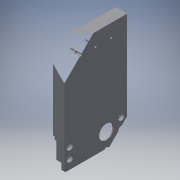
# Autodesk Inventor part: Base_motor_servo
Saved by Autodesk Inventor 2016 (Build 200138000, 138)
## iProperties
Created: 2018-05-05
Part Number: Base_motor_servo
Material: Genérico
Document SubType Name: Modeling
Designer: Innovacion Creativa
Density: 1 g/cm^3
Appearance: Valor por defecto
Author: Innovacion Creativa
Autodesk Inventor part; units mm, degrees
ref_plane "YZ Plane" through (0, 0, 0) normal (1, 0, 0) x (0, 1, 0)
ref_plane "XZ Plane" through (0, 0, 0) normal (0, 1, 0) x (-1, 0, 0)
ref_plane "XY Plane" through (0, 0, 0) normal (0, 0, 1) x (1, 0, 0)
sketch "Boceto2" plane through (0, 0, 0) normal (1, 0, 0) x (0, 1, 0)
  line L0 (44.4327, 14) -> (-16.1673, 14)
  line L1 (-16.1673, 14) -> (-16.1673, -14)
  line L2 (-16.1673, -14) -> (44.4327, -14)
  line L3 (44.4327, -14) -> (44.4327, 14)
  line L4 (-13.1673, 3.75) -> (-13.1673, -3.75) construction
  line L5 (41.4327, 3.75) -> (41.4327, -3.75) construction
  circle A0 centre (24.4327, 0) radius 6.4 construction
  circle A1 centre (24.4327, 0) radius 6.9
  point P0 (-16.1673, 0)
  point P1 (0, 0)
  dimension "d11" = 28
  dimension "d12" = 3
  dimension "d13" = 3
  dimension "d14" = 0.5
  constraints: 8 end point, 2 parallel, 1 centre point, 1 horizontal, 1 horizontal alignment, 1 midpoint, 1 perpendicular, 1 other
  measures "d11" distance of L0.end L1.end
  measures "d12" distance between parallel lines of L1 L4
  measures "d13" distance between parallel lines of L3 L5
  measures "d14" radial gap between concentric circles of A0 A1
extrude "Extrusión2" add sketch "Boceto2" along normal blind 1
sketch "Boceto3" plane through (0, 0, 0) normal (-1, 0, 0) x (0, 0, 1)
  line L0 (-8.9, 13.0341) -> (-1.9183, 13.0341) construction
  line L1 (-8.9, 1.5341) -> (-8.9, 13.0341) construction
  arc A0 (-8.9, 1.5341) -> (-7.9, 0.5341) centre (-7.9, 1.5341) ccw construction
  line L2 (7.9, 0.5341) -> (-7.9, 0.5341) construction
  arc A1 (7.9, 0.5341) -> (8.9, 1.5341) centre (7.9, 1.5341) ccw construction
  line L3 (8.9, 13.0341) -> (8.9, 1.5341) construction
  arc A2 (1.9183, 13.0341) -> (-1.9183, 13.0341) centre (0, 13.3841) ccw construction
  line L4 (1.9183, 13.0341) -> (8.9, 13.0341) construction
  line L5 (-8.9, 13.5341) -> (-2.8775, 13.5341)
  arc A3 (2.3898, 13.924) -> (-2.3898, 13.924) centre (0, 13.3841) ccw
  line L6 (2.8775, 13.5341) -> (8.9, 13.5341)
  line L7 (9.4, 13.0341) -> (9.4, 1.5341)
  arc A4 (7.9, 0.0341) -> (9.4, 1.5341) centre (7.9, 1.5341) ccw
  line L8 (7.9, 0.0341) -> (-7.9, 0.0341)
  arc A5 (-9.4, 1.5341) -> (-7.9, 0.0341) centre (-7.9, 1.5341) ccw
  line L9 (-9.4, 1.5341) -> (-9.4, 13.0341)
  arc A6 (-2.8775, 13.5341) -> (-2.3898, 13.924) centre (-2.8775, 14.0341) ccw
  arc A7 (2.3898, 13.924) -> (2.8775, 13.5341) centre (2.8775, 14.0341) ccw
  arc A8 (9.4, 13.0341) -> (8.9, 13.5341) centre (8.9, 13.0341) ccw
  arc A9 (-8.9, 13.5341) -> (-9.4, 13.0341) centre (-8.9, 13.0341) ccw
  point P0 (-2.4454, 13.5341)
  point P1 (2.4454, 13.5341)
  dimension "d19" = 0.5
  dimension "d20" = 0.5
  constraints: 16 point on circle, 10 end point, 8 tangent, 7 centre point, 3 equal radius, 2 point on line, 7 other
  measures "d19" distance between parallel lines of L1 L9
  measures "d20" radius of A6
extrude "Extrusión3" cut sketch "Boceto3" against normal blind 0.5
sketch "Boceto4" plane through (0, 0, 0) normal (-1, 0, 0) x (0, 0, 1)
  arc A0 (-4.7, 0.5341) -> (4.7, 0.5341) centre (0, 4.4546) ccw construction
  line L0 (-4.7, 0.5341) -> (-7.9, 0.5341) construction
  arc A1 (-8.9, 1.5341) -> (-7.9, 0.5341) centre (-7.9, 1.5341) ccw construction
  line L1 (-8.9, 1.5341) -> (-8.9, 20.8341) construction
  arc A2 (8.9, 20.8341) -> (-8.9, 20.8341) centre (0, 24.4327) ccw construction
  line L2 (8.9, 20.8341) -> (8.9, 13.0341) construction
  arc A3 (7.9, 0.5341) -> (8.9, 1.5341) centre (7.9, 1.5341) ccw construction
  line L3 (8.9, 13.0341) -> (8.9, 1.5341) construction
  line L4 (7.9, 0.5341) -> (4.7, 0.5341) construction
  arc A4 (-4.9437, 0) -> (4.9437, 0) centre (0, 4.4546) ccw
  line L5 (-4.9437, 0) -> (-7.9, 0)
  arc A5 (-9.4341, 1.5341) -> (-7.9, 0) centre (-7.9, 1.5341) ccw
  line L6 (-9.4341, 1.5341) -> (-9.4341, 20.7317)
  arc A6 (9.4341, 20.7317) -> (-9.4341, 20.7317) centre (0, 24.4327) ccw
  line L7 (9.4341, 20.7317) -> (9.4341, 13.0341)
  line L8 (9.4341, 13.0341) -> (9.4341, 1.5341)
  arc A7 (7.9, 0) -> (9.4341, 1.5341) centre (7.9, 1.5341) ccw
  line L9 (7.9, 0) -> (4.9437, 0)
  line L10 (14, 44.4327) -> (14, -16.1673)
  line L11 (14, -16.1673) -> (-14, -16.1673)
  line L12 (-14, -16.1673) -> (-14, 44.4327)
  line L13 (-14, 44.4327) -> (14, 44.4327)
  point P0 (0, 0)
extrude "Extrusión4" add sketch "Boceto4" along normal blind 2
sketch "Boceto5" plane through (-2, 0, 0) normal (-1, 0, 0) x (0, 0, 1)
  line L0 (0.6, -6.1673) -> (0.6, -13.1673) construction
  line L1 (-0.6, -6.1673) -> (-0.6, -13.1673) construction
  arc A0 (6.25, -12.5673) -> (3.75, -12.5673) centre (5, -10.7569) ccw construction
  arc A1 (-3.75, -12.5673) -> (-6.25, -12.5673) centre (-5, -10.7569) ccw construction
  line L2 (3.75, -13.1673) -> (-3.75, -13.1673) construction
  line L3 (8.9469, -6.6552) -> (8.9469, -13.7569)
  line L4 (7.9469, -14.7569) -> (-7.9469, -14.7569)
  line L5 (-8.9469, -13.7569) -> (-8.9469, -6.6552)
  line L6 (0.8, -13.6673) -> (0.8, -6.6552)
  line L7 (-0.8, -13.6673) -> (-0.8, -6.6552)
  line L8 (0.8, -13.1673) -> (-0.8, -13.1673) construction
  circle A2 centre (5, -10.7569) radius 1.75
  circle A3 centre (-5, -10.7569) radius 1.75
  circle A4 centre (0, 24.4327) radius 6.9 projected
  line L9 (14, 44.4327) -> (14, -16.1673) projected
  line L10 (14, -16.1673) -> (-14, -16.1673) projected
  line L11 (-14, -16.1673) -> (-14, 44.4327) projected
  line L12 (-14, 44.4327) -> (14, 44.4327) projected
  line L13 (-8.9, -6.1552) -> (8.9, -6.1552) construction
  line L14 (0.8, -13.6673) -> (-0.8, -13.6673)
  line L15 (8.9469, -6.6552) -> (0.8, -6.6552)
  line L16 (-0.8, -6.6552) -> (-8.9469, -6.6552)
  arc A5 (7.9469, -14.7569) -> (8.9469, -13.7569) centre (7.9469, -13.7569) ccw
  arc A6 (-8.9469, -13.7569) -> (-7.9469, -14.7569) centre (-7.9469, -13.7569) ccw
  line L17 (14, 44.4327) -> (14, -16.1673) projected
  line L18 (14, 14.1327) -> (-14, 14.1327) construction
  line L19 (-14, -16.1673) -> (-14, 44.4327) projected
  line L20 (8.9469, 34.9207) -> (8.9469, 42.0224)
  line L21 (7.9469, 43.0224) -> (-7.9469, 43.0224)
  line L22 (-8.9469, 42.0224) -> (-8.9469, 34.9207)
  line L23 (0.8, 41.9327) -> (0.8, 34.9207)
  line L24 (-0.8, 41.9327) -> (-0.8, 34.9207)
  circle A7 centre (5, 39.0224) radius 1.75
  circle A8 centre (-5, 39.0224) radius 1.75
  line L25 (0.8, 41.9327) -> (-0.8, 41.9327)
  line L26 (8.9469, 34.9207) -> (0.8, 34.9207)
  line L27 (-0.8, 34.9207) -> (-8.9469, 34.9207)
  arc A9 (8.9469, 42.0224) -> (7.9469, 43.0224) centre (7.9469, 42.0224) ccw
  arc A10 (-7.9469, 43.0224) -> (-8.9469, 42.0224) centre (-7.9469, 42.0224) ccw
  line L28 (8.9469, -13.7569) -> (8.9469, -14.7569)
  line L29 (8.9469, -14.7569) -> (7.9469, -14.7569)
  line L30 (8.9469, 42.0224) -> (8.9469, 43.0224)
  line L31 (8.9469, 43.0224) -> (7.9469, 43.0224)
  line L32 (7.9469, -14.7569) -> (8.9469, -13.7569)
  line L33 (8.9469, 42.0224) -> (7.9469, 43.0224)
  point P0 (0, 0)
  point P1 (0, -14.7569)
  point P2 (0, -13.1673)
  point P3 (8.9469, -6.1538)
  dimension "d26" = 0.2
  dimension "d27" = 3.5
  dimension "d28" = 3.5
  dimension "d30" = 4
  dimension "d31" = 0.5
  dimension "d32" = 0.5
  dimension "d33" = 1
  constraints: 48 end point, 14 symmetric about line, 9 point on circle, 8 centre point, 7 point on line, 5 midpoint, 5 tangent, 3 perpendicular, 2 coincident, 2 vertical, 2 vertical alignment, 1 equal radius, 1 horizontal, 1 horizontal alignment, 1 parallel, 5 other
  measures "d26" distance between parallel lines of L7 L1
  measures "d27" diameter of A2
  measures "d28" diameter of A3
  measures "d30" distance from line of L4 A0.centre
  measures "d31" distance between parallel lines of L14 L2
  measures "d32" distance between parallel lines of L13 L15
  measures "d33" radius of A5
extrude "Extrusión5" add sketch "Boceto5" along normal blind 6.2 contours L3 L32 L4 A6 L5 L16 L7 L14 L6 L15 | A5 L32 | L26 L23 L25 L24 L27 L22 A10 L21 L33 L20 | L33 A9
sketch "Boceto10" plane through (1, 0, 0) normal (1, 0, 0) x (0, 0, -1)
  line L0 (-36.5, -8.2479) -> (-36.5, 49.1121) construction
  circle A0 centre (0, 24.4327) radius 0.8 construction
  circle A1 centre (14.6, 24.4327) radius 1.6
  arc A2 (14.6, 19.8327) -> (14.6, 29.0327) centre (14.6, 24.4327) ccw
  line L1 (14.6, 29.0327) -> (10, 29.0327)
  line L2 (14.6, 19.8327) -> (10, 19.8327)
  line L3 (0, 29.0327) -> (0, 19.8327) construction
  line L4 (10, 29.0327) -> (10, 19.8327)
  circle A3 centre (-14.6, 24.4327) radius 1.6
  arc A4 (-14.6, 29.0327) -> (-14.6, 19.8327) centre (-14.6, 24.4327) ccw
  line L5 (-14.6, 29.0327) -> (-10, 29.0327)
  line L6 (-14.6, 19.8327) -> (-10, 19.8327)
  line L7 (-10, 29.0327) -> (-10, 19.8327)
  line L8 (14.6, 24.4327) -> (-14.6, 24.4327) construction
  point P0 (0, 0)
  point P1 (19.2, 24.4327)
  point P2 (19.2, 24.4327)
  dimension "d50" = 3.2
  dimension "d51" = 3
  dimension "d57" = 9.2
  dimension "d58" = 20
  constraints: 16 end point, 6 point on circle, 5 centre point, 5 symmetric about line, 2 horizontal, 2 horizontal alignment, 2 midpoint, 2 tangent, 2 vertical, 1 coincident, 1 vertical alignment, 5 other
  measures "d50" diameter of A1
  measures "d51" radial gap between concentric circles of A1 A2
  measures "d57" distance from line of L4 point (19.2, 24.433)
  measures "d58" distance between parallel lines of L7 L4
extrude "Extrusión10" add sketch "Boceto10" against normal blind 3
fillet "Empalme3" radius 10 4 edges at (-0.5, 29.0327, -14) (-0.5, 19.8327, -14) (-0.5, 29.0327, 14) (-0.5, 19.8327, 14)
sketch "Boceto11" plane through (-2, 0, 0) normal (-1, 0, 0) x (0, 0, 1)
  arc A0 (-14, 25.916) -> (-14, 22.9495) centre (-14.6, 24.4327) ccw projected
  arc A1 (14, 22.9495) -> (14, 25.916) centre (14.6, 24.4327) ccw projected
  circle A2 centre (14.6, 24.4327) radius 1.6
  circle A3 centre (-14.6, 24.4327) radius 1.6
  point P0 (0, 0)
  constraints: 2 centre point, 2 coincident, 2 concentric
extrude "Extrusión11" cut sketch "Boceto11" against normal blind 10
sketch "Boceto13" plane through (-2, -10.7569, 5) normal (-1, 0, 0) x (0, 0, 1)
  circle A0 centre (0, 0) radius 1.75 projected
  circle A1 centre (-10, 0) radius 1.75 projected
  circle A2 centre (0, 49.7792) radius 1.75 projected
  circle A3 centre (-10, 49.7792) radius 1.75 projected
  point P0 (-5, 10.7569)
extrude "Extrusión13" cut sketch "Boceto13" against normal blind 2.5
sketch "Boceto14" plane through (1, 0, 0) normal (1, 0, 0) x (0, 0, -1)
  line L0 (14, 44.4327) -> (-14, 44.4327) projected
  line L1 (0, 44.4327) -> (-10, 44.4327)
  line L2 (-10, 44.4327) -> (10, 44.4327)
  line L3 (-10, 44.4327) -> (10, 44.4327)
  line L4 (10, 44.4327) -> (10, 54.4327)
  line L5 (10, 54.4327) -> (-10, 54.4327)
  line L6 (-10, 54.4327) -> (-10, 44.4327)
  point P0 (0, 0)
  point P1 (11, 44.4327)
  point P2 (-11, 44.4327)
  dimension "d69" = 10
  dimension "d70" = 20
  dimension "d71" = 20
  dimension "d72" = 10
  constraints: 12 end point, 2 parallel, 2 point on line, 1 horizontal, 1 midpoint, 1 perpendicular
  measures "d69" distance of L1.start L1.end
  measures "d70" distance of L1.end L2.end
  measures "d71" distance of L5.end L4.end
  measures "d72" distance of L4.end L3.end
extrude "Extrusión14" add sketch "Boceto14" against normal blind 3
fillet "Empalme6" radius 2 2 edges at (-0.5, 54.4327, 10) (-0.5, 54.4327, -10)
sketch "Boceto15" plane through (1, 0, 0) normal (1, 0, 0) x (0, 0, -1)
  circle A0 centre (0, 49.0257) radius 1.75
  line L0 (-8, 54.4327) -> (8, 54.4327) projected
  line L1 (0, 49.0257) -> (-10, 49.0257)
  line L2 (-10, 44.4327) -> (-10, 52.4327) projected
  line L3 (0, 54.4327) -> (0, 49.0257)
  point P0 (0, 0)
  dimension "d76" = 3.5
  dimension "d86" = 5.407
  constraints: 4 end point, 1 centre point, 1 horizontal, 1 midpoint, 1 point on line, 1 vertical
  measures "d76" diameter of A0
  measures "d86" distance of L3.start L1.start
extrude "Extrusión15" cut sketch "Boceto15" against normal blind 3
sketch "Boceto16" plane through (1, 0, 0) normal (1, 0, 0) x (0, 0, -1)
  circle A0 centre (-5.04, 39.0224) radius 3
  circle A1 centre (5, 39.0224) radius 3
  circle A2 centre (5, -10.7461) radius 3
  circle A3 centre (-5.04, -10.7461) radius 3
  point P0 (0, 0)
  dimension "d79" = 6
  dimension "d80" = 6
  dimension "d81" = 6
  dimension "d82" = 6
  constraints: 4 centre point
  measures "d79" diameter of A0
  measures "d80" diameter of A1
  measures "d81" diameter of A2
  measures "d82" diameter of A3
extrude "Extrusión16" cut sketch "Boceto16" against normal blind 3
sketch "Boceto17" plane through (1, 0, 0) normal (1, 0, 0) x (0, 0, -1)
  circle A0 centre (-14.6125, 24.4601) radius 1.75
  circle A1 centre (14.5801, 24.4601) radius 1.75
  point P0 (0, 0)
  dimension "d87" = 3.5
  dimension "d88" = 3.5
  constraints: 2 centre point
  measures "d87" diameter of A0
  measures "d88" diameter of A1
extrude "Extrusión17" cut sketch "Boceto17" against normal blind 10
sketch "Boceto19" plane through (-2, 0, 0) normal (-1, 0, 0) x (0, 0, 1)
  line L0 (8.9469, -6.6552) -> (8.9469, -13.7569) projected
  line L1 (8.9469, -6.6552) -> (8.9469, -13.7569)
  line L2 (14, -16.1673) -> (-14, -16.1673) projected
  line L3 (8.9469, -16.1673) -> (88.9469, -16.1673)
  line L4 (88.9469, -16.1673) -> (88.9469, 44.4871)
  line L5 (88.9469, 44.4871) -> (8.9469, 44.4871)
  line L6 (8.9469, 44.4871) -> (8.9469, -16.1673)
  point P0 (0, 0)
  dimension "d91" = 80
  constraints: 10 end point, 2 parallel, 1 horizontal, 1 perpendicular, 1 point on line
  measures "d91" distance of L5.end L4.end
extrude "Extrusión18" add sketch "Boceto19" along normal blind 8 and the other way blind 3
sketch "Boceto20" plane through (-2, 0, 0) normal (-1, 0, 0) x (0, 0, 1)
  line L0 (-14, 44.4327) -> (-10, 44.4327) projected
  line L1 (-10, 44.4327) -> (10.7664, 44.4327)
  line L2 (10.7664, 44.4327) -> (10.7664, 56.4243)
  line L3 (10.7664, 56.4243) -> (-10, 56.4243)
  line L4 (-10, 56.4243) -> (-10, 44.4327)
  point P0 (0, 0)
  constraints: 8 end point, 2 parallel, 1 horizontal, 1 perpendicular
extrude "Extrusión19" cut sketch "Boceto20" against normal blind 10
sketch "Boceto21" plane through (-2, 0, 0) normal (-1, 0, 0) x (0, 0, 1)
  line L0 (-14, 35.6041) -> (-19.9956, 35.6041)
  line L1 (-19.9956, 35.6041) -> (-19.9956, 13.2614)
  line L2 (-19.9956, 13.2614) -> (-14, 13.2614)
  line L3 (-14, 13.2614) -> (-14, 35.6041)
  point P0 (0, 0)
  constraints: 8 end point, 2 parallel, 1 horizontal, 1 perpendicular
extrude "Extrusión20" cut sketch "Boceto21" against normal blind 10
sketch "Boceto22" plane through (-2, 0, 0) normal (-1, 0, 0) x (0, 0, 1)
  line L0 (-7.9469, -14.7569) -> (7.9469, -14.7569) projected
  line L1 (7.9469, -14.7569) -> (8.9469, -13.2115)
  line L2 (8.9469, 44.4871) -> (8.9469, -16.1673) projected
  line L3 (8.9469, -14.7569) -> (7.9469, -14.7569)
  point P0 (0, 0)
  constraints: 4 end point, 2 point on line, 1 perpendicular
extrude "Extrusión21" add sketch "Boceto22" along normal blind 6.3 and the other way blind 3
fillet "Empalme7" radius 2 2 edges at (-0.5, 44.4327, -14) (-0.5, -16.1673, -14)
sketch "Boceto23" plane through (-10, 0, 0) normal (-1, 0, 0) x (0, 0, 1)
  line L0 (7.9, 0) -> (4.9437, 0) projected
  line L1 (9.9, 34.9207) -> (7.9, 34.9207)
  line L2 (8.9469, -6.6552) -> (0.8, -6.6552) projected
  line L3 (7.9, -6.6552) -> (11.9, -6.6552)
  line L4 (11.9, -6.6552) -> (11.9, 34.9207)
  line L5 (11.9, 34.9207) -> (7.9, 34.9207)
  line L6 (7.9, 34.9207) -> (7.9, -6.6552)
  point P0 (0, 0)
  dimension "d105" = 2
  dimension "d130" = 4
  constraints: 10 end point, 2 parallel, 1 horizontal, 1 perpendicular, 1 point on line
  measures "d105" distance of L1.end L1.start
  measures "d130" distance of L5.end L4.end
extrude "Extrusión22" cut sketch "Boceto23" against normal blind 10.3
sketch "Boceto24" plane through (-10, 0, 0) normal (-1, 0, 0) x (0, 0, 1)
  line L0 (88.9469, 44.4871) -> (88.9469, -16.1673) projected
  line L1 (88.9469, -16.1673) -> (88.9469, 44.4871)
  line L2 (88.9469, 44.4871) -> (88.9469, 14.1599)
  line L3 (88.9469, -16.1673) -> (88.9469, 0)
  line L4 (88.9469, 14.1599) -> (88.9469, 29.3235)
  line L5 (88.9469, 0) -> (76.4469, 0)
  line L6 (88.9469, 29.3235) -> (76.4469, 29.3235)
  circle A0 centre (76.4469, 0) radius 1
  circle A1 centre (76.4469, 29.3235) radius 1
  line L7 (88.9469, 14.1599) -> (76.4469, 14.1599)
  circle A2 centre (76.4469, 14.1599) radius 1
  point P0 (0, 0)
  dimension "d108" = 12.5
  dimension "d109" = 12.5
  dimension "d110" = 2
  dimension "d111" = 2
  dimension "d112" = 12.5
  dimension "d113" = 2
  constraints: 14 end point, 3 centre point, 3 coincident, 2 midpoint, 2 perpendicular, 1 collinear, 1 horizontal, 1 point on line
  measures "d108" distance of L3.end L5.end
  measures "d109" distance of L4.end L6.end
  measures "d110" diameter of A0
  measures "d111" diameter of A1
  measures "d112" distance of L2.end L7.end
  measures "d113" diameter of A2
extrude "Extrusión23" cut sketch "Boceto24" against normal blind 5
sketch "Boceto25" plane through (1, 0, 0) normal (1, 0, 0) x (0, 0, -1)
  line L0 (-88.9469, -16.1673) -> (-88.9469, 44.4871) projected
  line L1 (-88.9469, 14.1599) -> (-76.4469, 14.1599)
  line L2 (-88.9469, 44.4871) -> (-88.9469, 14.1599)
  circle A0 centre (-76.4469, 29.3235) radius 1 projected
  line L3 (-88.9469, 29.3235) -> (-76.4469, 29.3235)
  line L4 (-88.9469, 14.1599) -> (-88.9469, 1.6599)
  line L5 (-88.9469, 1.6599) -> (-76.5855, 1.6599)
  circle A1 centre (-76.4469, 29.3235) radius 1
  circle A2 centre (-76.5855, 1.6599) radius 1
  circle A3 centre (-76.4469, 0) radius 1 projected
  circle A4 centre (-76.4469, 0) radius 1
  circle A5 centre (-76.4469, 14.1599) radius 1
  point P0 (0, 0)
  dimension "d116" = 12.5
  dimension "d117" = 12.5
  dimension "d118" = 12.5
  dimension "d121" = 2
  constraints: 10 end point, 4 centre point, 4 coincident, 2 horizontal, 2 midpoint, 1 collinear, 1 concentric, 1 perpendicular, 1 point on line
  measures "d116" distance of L1.start L1.end
  measures "d117" distance of L3.start L3.end
  measures "d118" distance of L1.start L4.end
  measures "d121" diameter of A5
extrude "Extrusión24" cut sketch "Boceto25" against normal blind 5 contours A0 | A5 | A3 A2 | A2 A3 picked at (-76.5506, 0.7735) picked at (-76.4878, -0.4416)
sketch "Boceto26" plane through (-10, 44.4871, 88.9469) normal (0, 1, 0) x (1, 0, 0)
  line L0 (11, 0) -> (0, 0) projected
  line L1 (5.5, 0) -> (5.5, 12.5)
  circle A0 centre (5.5, 12.5) radius 1
  point P0 (10, 88.9469)
  dimension "d122" = 12.5
  dimension "d123" = 2
  constraints: 2 end point, 1 centre point, 1 coincident, 1 midpoint, 1 vertical
  measures "d122" distance of L1.start L1.end
  measures "d123" diameter of A0
extrude "Extrusión25" cut sketch "Boceto26" against normal blind 5
sketch "Boceto27" plane through (-10, -16.1673, 88.9469) normal (0, -1, 0) x (1, 0, 0)
  line L0 (11, 0) -> (0, 0) projected
  line L1 (5.5, 0) -> (5.5, -12.5)
  circle A0 centre (5.5, -12.5) radius 1
  point P0 (10, -88.9469)
  dimension "d126" = 12.5
  dimension "d127" = 2
  constraints: 2 end point, 1 centre point, 1 coincident, 1 midpoint, 1 vertical
  measures "d126" distance of L1.start L1.end
  measures "d127" diameter of A0
extrude "Extrusión26" cut sketch "Boceto27" against normal blind 5
sketch "Boceto28" plane through (-10, 0, 0) normal (-1, 0, 0) x (0, 0, 1)
  line L0 (11.9, -6.6552) -> (8.9469, -6.6552) projected
  line L1 (8.9469, -6.6552) -> (8.9469, -16.1673) projected
  line L2 (11.9, -6.6552) -> (8.9469, -6.6552)
  line L3 (8.9469, -6.6552) -> (8.9469, -16.1673)
  line L4 (8.9469, -16.1673) -> (11.9, -16.1673)
  line L5 (11.9, -16.1673) -> (11.9, -6.6552)
  line L6 (8.9469, 44.4871) -> (8.9469, 34.9207) projected
  line L7 (8.9469, 34.9207) -> (11.9, 34.9207)
  line L8 (11.9, 34.9207) -> (11.9, 44.4871)
  line L9 (11.9, 44.4871) -> (8.9469, 44.4871)
  line L10 (8.9469, 44.4871) -> (8.9469, 34.9207)
  point P0 (0, 0)
  constraints: 16 end point, 4 parallel, 2 horizontal, 2 perpendicular, 1 point on line
extrude "Extrusión27" cut sketch "Boceto28" against normal blind 1.8
fillet "Empalme8" radius 1 1 edges at (-10, 14.1599, 11.9)
equation "\"d12\" = d13"
